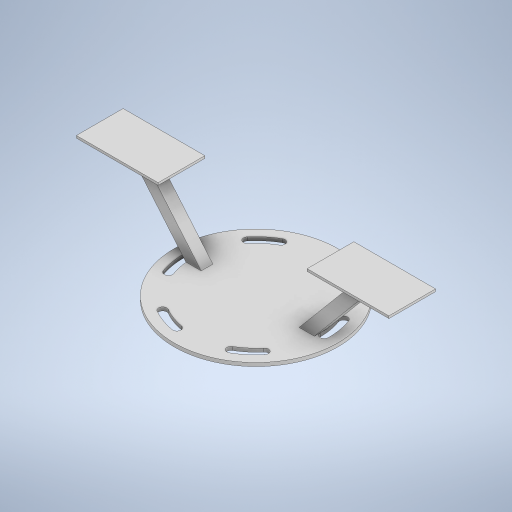
# Autodesk Inventor part: Bottom_plate
Saved by Autodesk Inventor 2024.3 (Build 283343000, 343)
## iProperties
Created: 2025-03-09
Part Number: Bottom_plate
Material: Generic
Document SubType Name: Modeling
Designer: ajclo
Density: 1 g/cm^3
Appearance: Default
Author: ajclo
Autodesk Inventor part; units mm, degrees
ref_plane "YZ Plane" through (0, 0, 0) normal (1, 0, 0) x (0, 1, 0)
ref_plane "XZ Plane" through (0, 0, 0) normal (0, 1, 0) x (-1, 0, 0)
ref_plane "XY Plane" through (0, 0, 0) normal (0, 0, 1) x (1, 0, 0)
sketch "Sketch1" plane through (0, 0, 0) normal (0, 1, 0) x (-1, 0, 0)
  circle A0 centre (0, 0) radius 70
  dimension "d0" = 140
  constraints: 1 centre point, 1 coincident
  measures "d0" diameter of A0
extrude "Extrusion1" add sketch "Sketch1" along normal blind 3
sketch "Sketch2" plane through (0, 3, 0) normal (0, 1, 0) x (1, 0, 0)
  circle A0 centre (0, 0) radius 62
  circle A1 centre (0, 0) radius 55
  arc A2 (-55, 0) -> (-62, 0) centre (-58.5, 0) ccw
  arc A3 (-58.2641, -21.1966) -> (-51.6859, -18.8034) centre (-54.975, -20) ccw
  dimension "d3" = 124
  dimension "d4" = 110
  dimension "d7" = 20
  constraints: 8 point on circle, 4 centre point, 4 tangent, 2 coincident
  measures "d3" diameter of A0
  measures "d4" diameter of A1
  measures "d7" vertical distance of point (0, 0) A3.centre
extrude "Extrusion2" cut sketch "Sketch2" against normal through all contours A2 A1 A3 A0 picked at (-56.7601, -18.0974)
pattern_circular "Circular Pattern1" count 6 over 360 about axis through (0, 0, 0) along (0, 1, 0) of "Extrusion2"
sketch "Sketch4" plane through (0, 0, 0) normal (0, 0, 1) x (1, 0, 0)
  line L0 (70, 3) -> (-70, 3) projected
  line L1 (-41.9459, 3) -> (-92.2919, 63)
  line L2 (-92.2919, 63) -> (-105.346, 63)
  line L3 (-105.346, 63) -> (-55, 3)
  point P0 (0, 0)
  point P1 (0, 3)
  dimension "d13" = 50
  dimension "d14" = 60
  dimension "d15" = 55
  dimension "d16" = 10
  constraints: 6 end point, 2 parallel, 2 point on line, 1 midpoint
  measures "d13" angle of L0 L1
  measures "d14" vertical distance of L1.start L1.end
  measures "d15" distance of point (0, 3) L3.end
  measures "d16" distance between parallel lines of L3 L1
extrude "Extrusion3" add sketch "Sketch4" along normal mid plane 10
mirror "Mirror1" about plane through (0, 0, 0) normal (1, 0, 0) of "Extrusion3"
sketch "Sketch6" plane through (0, 0, 0) normal (0, 0, 1) x (1, 0, 0)
  line L0 (-63.8189, 65) -> (-133.8189, 65)
  line L1 (-133.8189, 65) -> (-133.8189, 63)
  line L2 (-133.8189, 63) -> (-63.8189, 63)
  line L3 (-63.8189, 63) -> (-63.8189, 65)
  line L4 (-63.8189, 65) -> (-133.8189, 63) construction
  line L5 (-133.8189, 65) -> (-63.8189, 63) construction
  line L6 (-105.346, 63) -> (-92.2919, 63) projected
  point P0 (0, 0)
  point P1 (-98.8189, 64)
  point P2 (-98.8189, 63)
  point P3 (-98.8189, 63)
  dimension "d22" = 2
  dimension "d23" = 70
  dimension "d24" = 0
  constraints: 12 end point, 4 midpoint, 2 parallel, 1 collinear, 1 horizontal, 1 perpendicular
  measures "d22" distance of L0.end L1.end
  measures "d23" distance of L0.start L0.end
  measures "d24" distance of point (-98.819, 63) point (-98.819, 63)
extrude "Extrusion4" add sketch "Sketch6" along normal mid plane 40
mirror "Mirror2" about plane through (0, 0, 0) normal (1, 0, 0) of "Extrusion4"
body "Solid1"
